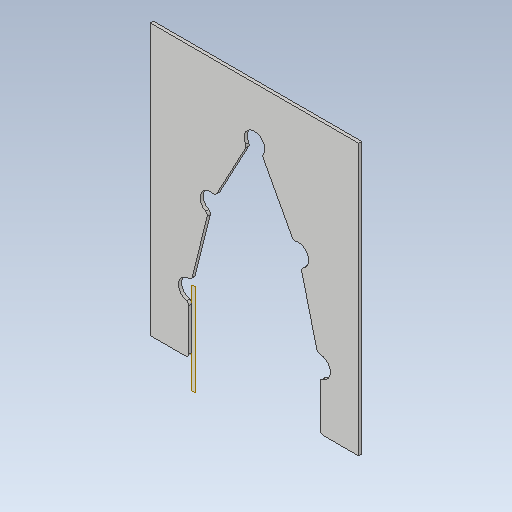
# Autodesk Inventor part: svejselære 1
Saved by Autodesk Inventor 2020.1 (Build 241239000, 239)
## iProperties
Created: 2019-10-09
Part Number: svejselære 1
Material: Generic
Document SubType Name: Sheet Metal
Designer: loppen
Density: 1 g/cm^3
Sheet Metal Rule: Default_mm
Appearance: Default
Flat Pattern Width: 20 cm
Flat Pattern Length: 26 cm
Flat Pattern Area: 520 cm^2
Sheet Metal Width: 200,000 mm
Sheet Metal Length: 260,000 mm
Sheet Metal Area: 52000,000 mm^2
Author: loppen
Autodesk Inventor part; units mm, degrees
ref_plane "YZ Plane" through (0, 0, 0) normal (1, 0, 0) x (0, 1, 0)
ref_plane "XZ Plane" through (0, 0, 0) normal (0, 1, 0) x (-1, 0, 0)
ref_plane "XY Plane" through (0, 0, 0) normal (0, 0, 1) x (1, 0, 0)
ref_plane "Work Plane1" through (0, 0, 0) normal (0, 0, 1) x (1, 0, 0)
sketch "Sketch1" plane through (0, 0, 0) normal (0, 0, 1) x (1, 0, 0)
  line L0 (60, 154.3122) -> (60, -124.8582) construction
  line L1 (-40, -55.6878) -> (-40, 204.3122)
  line L2 (-40, 204.3122) -> (160, 204.3122)
  line L3 (160, 204.3122) -> (160, -55.6878)
  arc A0 (-2.8578, 10.3642) -> (-5.2959, -9.3561) centre (-2.949, 0.3646) ccw
  arc A1 (20.3319, 92.7038) -> (13.1645, 74.1711) centre (17.8081, 83.0275) ccw
  arc A2 (68.5267, 149.0877) -> (51.4733, 149.0877) centre (60, 154.3122) ccw
  arc A3 (106.8355, 74.1711) -> (99.6681, 92.7038) centre (102.1919, 83.0275) ccw
  arc A4 (125.2959, -9.3561) -> (122.8578, 10.3642) centre (122.949, 0.3646) ccw
  line L4 (-3, -12.2723) -> (-3, -52.6878)
  line L5 (0.0792, 12.6334) -> (14.681, 70.7835)
  line L6 (23.7332, 94.1894) -> (51.5594, 146.1031)
  line L7 (68.4406, 146.1031) -> (96.2668, 94.1894)
  line L8 (105.319, 70.7835) -> (119.9208, 12.6334)
  line L9 (123, -12.2723) -> (123, -52.6878)
  line L10 (160, -55.6878) -> (126, -55.6878)
  line L11 (-6, -55.6878) -> (-40, -55.6878)
  line L12 (-3, -0.4636) -> (-3, -80.75)
  line L13 (17.557, 82.2366) -> (-2.7968, 1.1803)
  line L14 (54.0507, 150.7511) -> (18.1545, 83.7816)
  line L15 (101.8455, 83.7816) -> (65.9493, 150.7511)
  line L16 (122.7968, 1.1803) -> (102.443, 82.2366)
  line L17 (123, -80.75) -> (123, -0.4636)
  arc A5 (-2.7968, 1.1803) -> (-3, -0.4636) centre (3.75, -0.4636) ccw
  arc A6 (18.1545, 83.7816) -> (17.557, 82.2366) centre (24.1037, 80.5927) ccw
  arc A7 (65.9493, 150.7511) -> (54.0507, 150.7511) centre (60, 147.5622) ccw
  arc A8 (102.443, 82.2366) -> (101.8455, 83.7816) centre (95.8963, 80.5927) ccw
  arc A9 (123, -0.4636) -> (122.7968, 1.1803) centre (116.25, -0.4636) ccw
  line L18 (60, 147.5622) -> (60, 430.3186) construction
  arc A10 (-6, -55.6878) -> (-3, -52.6878) centre (-6, -52.6878) ccw
  arc A11 (-3, -12.2723) -> (-5.2959, -9.3561) centre (-6, -12.2723) ccw
  arc A12 (-2.8578, 10.3642) -> (0.0792, 12.6334) centre (-2.8305, 13.3641) ccw
  arc A13 (14.681, 70.7835) -> (13.1645, 74.1711) centre (11.7714, 71.5142) ccw
  arc A14 (20.3319, 92.7038) -> (23.7332, 94.1894) centre (21.089, 95.6067) ccw
  arc A15 (51.5594, 146.1031) -> (51.4733, 149.0877) centre (48.9153, 147.5204) ccw
  arc A16 (68.5267, 149.0877) -> (68.4406, 146.1031) centre (71.0847, 147.5204) ccw
  arc A17 (96.2668, 94.1894) -> (99.6681, 92.7038) centre (98.911, 95.6067) ccw
  arc A18 (106.8355, 74.1711) -> (105.319, 70.7835) centre (108.2286, 71.5142) ccw
  arc A19 (119.9208, 12.6334) -> (122.8578, 10.3642) centre (122.8305, 13.3641) ccw
  arc A20 (125.2959, -9.3561) -> (123, -12.2723) centre (126, -12.2723) ccw
  arc A21 (123, -52.6878) -> (126, -55.6878) centre (126, -52.6878) ccw
  point P0 (0, 0)
  point P1 (-0.563, 10.0758)
  point P2 (-3, -9.6353)
  point P3 (22.4874, 91.8652)
  point P4 (15.3233, 73.3412)
  point P5 (67.5532, 147.7587)
  point P6 (52.4468, 147.7587)
  point P7 (104.6767, 73.3412)
  point P8 (97.5126, 91.8652)
  point P9 (123, -9.6353)
  point P10 (120.563, 10.0758)
  point P11 (97.5126, 91.8652)
  point P12 (123, -55.6878)
  point P13 (123, -55.6878)
  point P14 (-3, -55.6878)
  dimension "d0" = 200
  dimension "d1" = 100
  dimension "d2" = 260
  dimension "d3" = 50
  dimension "d4" = 10
  dimension "d5" = 10
  dimension "d6" = 10
  dimension "d7" = 10
  dimension "d8" = 10
  dimension "d9" = 3
  measures "d0" distance of L1.end L2.end
  measures "d1" distance between parallel lines of L1 L0
  measures "d2" distance of L1.start L1.end
  measures "d3" distance from line of L0.start L2
  measures "d4" radius of A0
  measures "d5" radius of A1
  measures "d6" radius of A2
  measures "d7" radius of A3
  measures "d8" radius of A4
  measures "d9" radius of A10
extrude "Plate1" add sketch "Sketch1" along normal blind 3 contours L1 L2 L3 L10 A21 L9 A20 A4 A19 L8 A18 A3 A17 L7 A16 A2 A15 L6 A14 A1 A13 L5 A12 A0 A11 L4 A10 L11
equation "\"d1\" = 0.5 * d0"
equation "\"d5\" = d4"
equation "\"d6\" = d4"
equation "\"d7\" = d4"
equation "\"d8\" = d4"
equation "\"d10\" = Thickness"
equation "\"BendRadius\" = Thickness"
equation "\"BendReliefWidth\" = Thickness"
equation "\"BendReliefDepth\" = 0.5 * Thickness"
equation "\"CornerReliefSize\" = 4 * Thickness"
equation "\"MinimumRemnant\" = 2 * Thickness"
equation "\"TransitionRadius\" = BendRadius"
equation "\"JacobiRadiusSize\" = BendRadius"
equation "\"GapSize\" = Thickness"
equation "\"Thickness\" = 3"
body "Solid1"
